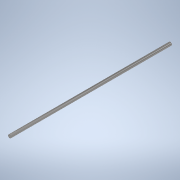
# Autodesk Inventor part: HeadTube
Saved by Autodesk Inventor 2020 (Build 240168000, 168)
## iProperties
Created: 2020-03-07
Part Number: HeadTube
Material: Stainless Steel, Austenitic
Document SubType Name: Modeling
Designer: 10300812
Density: 8 g/cm^3
Appearance: Semi-Polished
Mass: 43.9823 g
Surface Area: 110.396 cm^2
Volume: 5.49779 cm^3
Author: 10300812
Autodesk Inventor part; units mm, degrees
ref_plane "YZ Plane" through (0, 0, 0) normal (1, 0, 0) x (0, 1, 0)
ref_plane "XZ Plane" through (0, 0, 0) normal (0, 1, 0) x (-1, 0, 0)
ref_plane "XY Plane" through (0, 0, 0) normal (0, 0, 1) x (1, 0, 0)
sketch "Sketch1" plane through (0, 0, 0) normal (0, 0, 1) x (1, 0, 0)
  circle A0 centre (0, 0) radius 1.25
  circle A1 centre (0, 0) radius 2.5
  dimension "d0" = 2.5
  dimension "d1" = 5
  constraints: 2 centre point, 2 coincident
  measures "d0" diameter of A0
  measures "d1" diameter of A1
extrude "Extrusion1" add sketch "Sketch1" along normal blind 55
body "Solid1"
